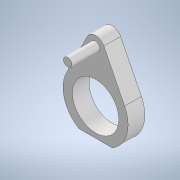
# Autodesk Inventor part: ClickSpringBacking
Saved by Autodesk Inventor 2021 (Build 250183000, 183)
## iProperties
Created: 2021-07-10
Part Number: ClickSpringBacking
Material: Generic
Document SubType Name: Modeling
Designer: teh18
Density: 1 g/cm^3
Appearance: Default
Author: teh18
Autodesk Inventor part; units mm, degrees
ref_plane "YZ Plane" through (0, 0, 0) normal (1, 0, 0) x (0, 1, 0)
ref_plane "XZ Plane" through (0, 0, 0) normal (0, 1, 0) x (-1, 0, 0)
ref_plane "XY Plane" through (0, 0, 0) normal (0, 0, 1) x (1, 0, 0)
sketch "Sketch1" plane through (0, 0, 0) normal (0, 0, 1) x (1, 0, 0)
  circle A0 centre (0, 0) radius 3.75 projected
  circle A1 centre (0, 0) radius 15 projected
  arc A2 (0, -15) -> (0, -15) centre (0, 0) ccw
  line L0 (44.9276, 33.0458) -> (45.2557, 31.8342) projected
  arc A3 (45.2557, 31.8342) -> (43.9307, 28.6117) centre (50, 28) ccw projected
  line L1 (43.9307, 28.6117) -> (42.8453, 27.9812) projected
  line L2 (42.8453, 27.9812) -> (43.934, 27.3564) projected
  arc A4 (43.934, 27.3564) -> (45.2759, 24.1409) centre (50, 28) ccw projected
  line L3 (45.2759, 24.1409) -> (44.9542, 22.9276) projected
  line L4 (44.9542, 22.9276) -> (46.1658, 23.2557) projected
  arc A5 (46.1658, 23.2557) -> (49.3883, 21.9307) centre (50, 28) ccw projected
  line L5 (49.3883, 21.9307) -> (50.0188, 20.8453) projected
  line L6 (50.0188, 20.8453) -> (50.6436, 21.934) projected
  arc A6 (50.6436, 21.934) -> (53.8591, 23.2759) centre (50, 28) ccw projected
  line L7 (53.8591, 23.2759) -> (55.0724, 22.9542) projected
  line L8 (55.0724, 22.9542) -> (54.7443, 24.1658) projected
  arc A7 (54.7443, 24.1658) -> (56.0693, 27.3883) centre (50, 28) ccw projected
  line L9 (56.0693, 27.3883) -> (57.1547, 28.0188) projected
  line L10 (57.1547, 28.0188) -> (56.066, 28.6436) projected
  arc A8 (56.066, 28.6436) -> (54.7241, 31.8591) centre (50, 28) ccw projected
  line L11 (54.7241, 31.8591) -> (55.0458, 33.0724) projected
  line L12 (55.0458, 33.0724) -> (53.8342, 32.7443) projected
  arc A9 (53.8342, 32.7443) -> (50.6117, 34.0693) centre (50, 28) ccw projected
  line L13 (50.6117, 34.0693) -> (49.9812, 35.1547) projected
  line L14 (49.9812, 35.1547) -> (49.3564, 34.066) projected
  arc A10 (49.3564, 34.066) -> (46.1409, 32.7241) centre (50, 28) ccw projected
  line L15 (46.1409, 32.7241) -> (44.9276, 33.0458) projected
  circle A11 centre (50, 28) radius 20 projected
  circle A12 centre (0, 28) radius 5
  line L16 (150, -15) -> (-20, -15) projected
  circle A13 centre (0, 0) radius 12.5
  line L17 (4.6702, 29.7857) -> (14.0107, 5.3571)
  line L18 (-14.0107, 5.3571) -> (-4.6702, 29.7857)
  dimension "d0" = 30
  dimension "d3" = 10
  dimension "d8" = 25
  constraints: 6 point on circle, 4 end point, 4 tangent, 3 centre point, 2 point on line, 1 coincident, 1 horizontal alignment, 1 vertical alignment
  measures "d0" diameter of A2
  measures "d3" diameter of A12
  measures "d8" diameter of A13
extrude "Extrusion1" add sketch "Sketch1" along normal blind 9 contours A1 | A1 L18 A12 L17 | A12
sketch "Sketch2" plane through (0, 0, 9) normal (0, 0, 1) x (1, 0, 0)
  circle A0 centre (0, 28) radius 2.25
  circle A1 centre (0, 28) radius 11
  line L0 (44.2385, 23.4259) -> (45.8503, 23.6652) projected
  arc A2 (45.8503, 23.6652) -> (48.5121, 22.1865) centre (50, 28) ccw projected
  line L1 (48.5121, 22.1865) -> (49.1604, 20.6917) projected
  line L2 (49.1604, 20.6917) -> (50.1308, 22.0006) projected
  arc A3 (50.1308, 22.0006) -> (53.0586, 22.8371) centre (50, 28) ccw projected
  line L3 (53.0586, 22.8371) -> (54.5741, 22.2385) projected
  line L4 (54.5741, 22.2385) -> (54.3348, 23.8503) projected
  arc A4 (54.3348, 23.8503) -> (55.8135, 26.5121) centre (50, 28) ccw projected
  line L5 (55.8135, 26.5121) -> (57.3083, 27.1604) projected
  line L6 (57.3083, 27.1604) -> (55.9994, 28.1308) projected
  arc A5 (55.9994, 28.1308) -> (55.1629, 31.0586) centre (50, 28) ccw projected
  line L7 (55.1629, 31.0586) -> (55.7615, 32.5741) projected
  line L8 (55.7615, 32.5741) -> (54.1497, 32.3348) projected
  arc A6 (54.1497, 32.3348) -> (51.4879, 33.8135) centre (50, 28) ccw projected
  line L9 (51.4879, 33.8135) -> (50.8396, 35.3083) projected
  line L10 (50.8396, 35.3083) -> (49.8692, 33.9994) projected
  arc A7 (49.8692, 33.9994) -> (46.9414, 33.1629) centre (50, 28) ccw projected
  line L11 (46.9414, 33.1629) -> (45.4259, 33.7615) projected
  line L12 (45.4259, 33.7615) -> (45.6652, 32.1497) projected
  arc A8 (45.6652, 32.1497) -> (44.1865, 29.4879) centre (50, 28) ccw projected
  line L13 (44.1865, 29.4879) -> (42.6917, 28.8396) projected
  line L14 (42.6917, 28.8396) -> (44.0006, 27.8692) projected
  arc A9 (44.0006, 27.8692) -> (44.8371, 24.9414) centre (50, 28) ccw projected
  line L15 (44.8371, 24.9414) -> (44.2385, 23.4259) projected
  circle A10 centre (50, 28) radius 18 projected
  point P0 (0, 0)
  dimension "d4" = 4.5
  dimension "d7" = 22
  constraints: 2 centre point, 2 coincident
  measures "d4" diameter of A0
  measures "d7" diameter of A1
extrude "Extrusion2" add sketch "Sketch2" along normal blind 15 contours A0
body "Solid1"
